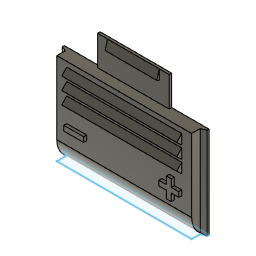
Battery Door (Autodesk Fusion 360 design; units mm, degrees)
Autodesk Fusion 360 part; units mm, degrees
sketch "sketch 1635" plane through (0, 0, -18.387) normal (0, 0, -1) x (1, 0, 0)
  line L0 (66.9, 86.8123) -> (66.9, 85.1)
  line L1 (66.9, 85.1) -> (65.9, 84.7123)
  line L2 (65.9, 84.7123) -> (65.9, 84.3123)
  line L3 (65.9, 84.3123) -> (80.461, 84.3123)
  line L4 (95.0219, 84.3123) -> (80.461, 84.3123)
  line L5 (95.0219, 84.7123) -> (95.0219, 84.3123)
  line L6 (94.0219, 85.1) -> (95.0219, 84.7123)
  line L7 (94.0219, 86.8123) -> (94.0219, 85.1)
  line L8 (66.9, 86.8123) -> (94.0219, 86.8123)
extrude "Extrude1" add sketch "sketch 1635" against normal up to surface (18.387 mm away)
sketch "Sketch7" plane through (0, 0, 0) normal (0, 0, 1) x (-1, 0, 0)
  line L0 (-95.0219, 84.3123) -> (-65.9, 84.3123)
  line L1 (-65.9, 84.3123) -> (-65.9, 84.7123)
  line L2 (-66.9, 86.8123) -> (-94.0219, 86.8123)
  line L3 (-116.01, 84.8123) -> (4.2372, 84.8123) construction
  line L4 (-95.0219, 84.3123) -> (-95.0219, 84.8123) construction
  line L5 (-87.5, 82.9623) -> (-73.1, 82.9623)
  line L6 (-73.1, 82.9623) -> (-73.1, 84.8123)
  line L7 (-73.1, 84.8123) -> (-87.5, 84.8123)
  line L8 (-87.5, 84.8123) -> (-87.5, 82.9623)
  line L9 (-65.9, 84.7123) -> (-66.9, 85.1)
  line L10 (-66.9, 85.1) -> (-66.9, 86.8123)
  line L11 (-94.0219, 86.8123) -> (-94.0219, 85.1)
  line L12 (-94.0219, 85.1) -> (-95.0219, 84.7123)
  line L13 (-95.0219, 84.7123) -> (-95.0219, 84.3123)
  constraint coincident L0.start L4.start
  constraint coincident L3 L4.end
  constraint perpendicular L3 L4
  constraint horizontal L5
  constraint vertical L6
  constraint horizontal L7
  constraint vertical L8
  constraint coincident L4.end L7
extrude "Extrude7" add sketch "Sketch7" along normal blind 6 contours L0 L6 L7 L8
sketch "Sketch8" plane through (87.5, 0, 0) normal (1, 0, 0) x (0, 1, 0)
  line L0 (-84.8123, 0) -> (-84.3123, 0)
  line L1 (-84.3123, 0) -> (-84.3123, 6)
  line L2 (-84.3123, 6) -> (-84.8123, 6)
  line L3 (-84.8123, 6) -> (-84.8123, 0)
  line L4 (-84.8123, 6) -> (-85.3123, 4.2426)
  line L5 (-85.3123, 4.2426) -> (-84.8123, 4)
  dimension "d558" = 0.5
  dimension "d559" = 2
  dimension "d560" = 100
  constraint coincident L2.end L3.start
  constraint coincident L3 L5.end
  measures "d558" distance of L3 L4.end
  measures "d559" distance of L2.end L5.end
  measures "d560" angle of L4 L5
extrude "Extrude8" add sketch "Sketch8" against normal up to surface (10.4 mm away) from surface at -2 contours L3 L4 L5
sketch "Sketch9" plane through (94.0219, 0, 0) normal (1, 0, 0) x (0, 1, 0)
  line L0 (-85.1, 0) -> (-86.8123, 0)
  line L1 (-86.8123, 0) -> (-86.8123, -18.387)
  line L2 (-86.8123, -18.387) -> (-85.1, -18.387)
  arc A0 (-86.8123, -14.6454) -> (-85.2027, -18.0944) centre (-82.3123, -14.6454) ccw
  line L3 (-86.8123, -18.387) -> (-86.8123, -14.6454)
  line L4 (-86.8123, 0) -> (-86.8123, -9.1935)
  line L5 (-86.8123, -1.0019) -> (-87.8123, -2.0656)
  line L6 (-87.8123, -2.0656) -> (-86.8123, -3.0057)
  line L7 (-87.8123, -4.5715) -> (-86.8123, -5.5116)
  line L8 (-86.8123, -3.5078) -> (-87.8123, -4.5715)
  line L9 (-87.8123, -7.0774) -> (-86.8123, -8.0175)
  line L10 (-86.8123, -6.0137) -> (-87.8123, -7.0774)
  line L11 (-86.8123, -18.387) -> (-86.8123, -18.5527)
  line L12 (-86.8123, -18.5527) -> (-84.815, -18.5526)
  line L13 (-84.815, -18.5526) -> (-84.815, -18.3852)
  ellipse E0 centre (-82.3123, -14.6454) end of major axis (-82.3123, -19.1454) minor radius 4.5 (-85.2027, -18.0944) -> (-84.815, -18.3852) ccw
  dimension "d565" = 1
  dimension "d568" = 0
  dimension "d569" = -7.5177
  constraint coincident L1.end L2.start
  constraint coincident A0.start L3.end
  constraint coincident L0.end L1.start
  constraint midpoint L1 L4.end
  constraint coincident L4 L5.start
  constraint perpendicular L5 L6
  constraint coincident L1 L6.end
  constraint perpendicular L11 L12
  constraint parallel L11 L13
  measures "d565" distance of L4 L5.end
extrude "Extrude9" add sketch "Sketch9" against normal up to surface (23.1219 mm away) from surface at -2
extrude "Extrude10" cut sketch "Sketch9" along normal up to surface (-28.1219 mm away) and the other way up to surface (-1 mm away) contours L1 A0 L3 L11 L12 L13 E0
sketch "Sketch10" plane through (0, -86.8123, 0) normal (0, -1, 0) x (1, 0, 0)
  line L0 (92.0219, -5.5116) -> (68.9, -5.5116)
  line L1 (68.9, -5.5116) -> (68.9, -3.5078)
  line L2 (68.9, -3.5078) -> (92.0219, -3.5078)
  line L3 (92.0219, -3.5078) -> (92.0219, -5.5116)
  line L4 (92.0219, -3.0057) -> (68.9, -3.0057)
  line L5 (68.9, -3.0057) -> (68.9, -1.0019)
  line L6 (68.9, -1.0019) -> (92.0219, -1.0019)
  line L7 (92.0219, -1.0019) -> (92.0219, -3.0057)
  line L8 (92.0219, -8.0175) -> (68.9, -8.0175)
  line L9 (68.9, -8.0175) -> (68.9, -6.0137)
  line L10 (68.9, -6.0137) -> (92.0219, -6.0137)
  line L11 (92.0219, -6.0137) -> (92.0219, -8.0175)
  line L12 (66.9, -14.6454) -> (94.0219, -14.6454)
  line L13 (94.0219, -14.6454) -> (94.0219, 0)
  line L14 (94.0219, 0) -> (66.9, 0)
  line L15 (66.9, 0) -> (66.9, -14.6454)
  line L16 (66.9, -8.0175) -> (94.0219, -8.0175) construction
  line L17 (80.461, -8.0175) -> (80.461, -14.6454) construction
  line L18 (80.461, -11.3314) -> (94.0219, -11.3314) construction
  line L19 (80.461, -11.3314) -> (66.9, -11.3314) construction
  line L20 (73.6805, -11.3314) -> (73.6805, -8.0175) construction
  line L21 (87.2415, -11.3314) -> (87.2415, -8.0175) construction
  line L22 (72.9, -11.3314) -> (72.9, -10.8314)
  line L23 (72.9, -10.8314) -> (68.9, -10.8314)
  line L24 (68.9, -10.8314) -> (68.9, -11.3314)
  line L25 (68.9, -11.8314) -> (68.9, -11.3314)
  line L26 (72.9, -11.8314) -> (68.9, -11.8314)
  line L27 (72.9, -11.3314) -> (72.9, -11.8314)
  line L28 (88.0219, -11.3314) -> (88.0219, -10.8314)
  line L29 (88.0219, -10.8314) -> (89.5219, -10.8314)
  line L30 (89.5219, -10.8314) -> (89.5219, -9.3314)
  line L31 (89.5219, -9.3314) -> (90.5219, -9.3314)
  line L32 (90.5219, -9.3314) -> (90.5219, -10.8314)
  line L33 (90.5219, -10.8314) -> (92.0219, -10.8314)
  line L34 (92.0219, -10.8314) -> (92.0219, -11.3314)
  line L35 (88.0219, -11.3314) -> (88.0219, -11.8314)
  line L36 (88.0219, -11.8314) -> (89.5219, -11.8314)
  line L37 (89.5219, -11.8314) -> (89.5219, -13.3314)
  line L38 (89.5219, -13.3314) -> (90.5219, -13.3314)
  line L39 (90.5219, -13.3314) -> (90.5219, -11.8314)
  line L40 (90.5219, -11.8314) -> (92.0219, -11.8314)
  line L41 (92.0219, -11.8314) -> (92.0219, -11.3314)
  dimension "d656" = 1
  dimension "d657" = 1
  dimension "d658" = 1.5
  dimension "d659" = 4
  dimension "d662" = 1.5
  dimension "d663" = 0.5
  dimension "d664" = 0.5
  dimension "d665" = 2
  constraint coincident L15 L16.start
  constraint coincident L13 L16.end
  constraint perpendicular L13 L16
  constraint midpoint L8 L17.start
  constraint midpoint L12 L17.end
  constraint midpoint L17 L18.start
  constraint coincident L13 L18.end
  constraint perpendicular L13 L18
  constraint coincident L15 L19.end
  constraint perpendicular L15 L19
  constraint midpoint L19 L20.start
  constraint perpendicular L16 L20
  constraint coincident L8 L20.end
  constraint midpoint L18 L21.start
  constraint perpendicular L18 L21
  constraint coincident L16 L17.start
  constraint coincident L19 L22.start
  constraint perpendicular L19 L22
  constraint perpendicular L22 L23
  constraint coincident L19 L24.end
  constraint perpendicular L19 L24
  constraint symmetric L19 L22.start L27.start
  constraint symmetric L19 L22.end L26.start
  constraint symmetric L19 L23.end L25.start
  constraint symmetric L19 L24.end L25.end
  constraint coincident L18 L28.start
  constraint perpendicular L18 L28
  constraint perpendicular L28 L29
  constraint perpendicular L29 L30
  constraint perpendicular L30 L31
  constraint perpendicular L31 L32
  constraint perpendicular L32 L33
  constraint coincident L18 L34.end
  constraint perpendicular L18 L34
  constraint symmetric L18 L28.start L35.start
  constraint symmetric L18 L28.end L35.end
  constraint symmetric L18 L29.end L36.end
  constraint symmetric L18 L30.end L37.end
  constraint symmetric L18 L31.end L38.end
  constraint symmetric L18 L32.end L39.end
  constraint symmetric L18 L33.end L40.end
  constraint symmetric L18 L34.end L41.end
  constraint collinear L9 L24
  constraint collinear L11 L34
  measures "d656" distance of L23 L26
  measures "d657" distance of L30.end L31.end
  measures "d658" distance of L32.end L33.end
  measures "d659" distance of L22.end L23.end
  measures "d662" distance of L28.end L29.end
  measures "d663" distance of L18 L33
  measures "d664" distance of L18 L29
  measures "d665" distance of L18 L31
extrude "Extrude11" add sketch "Sketch10" along normal blind 0.6 contours L22 L23 L24 L25 L26 L27 | L28 L29 L30 L31 L32 L33 L34 L35 L36 L37 L38 L39 L40 L41
